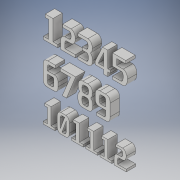
# Autodesk Inventor part: Number
Saved by Autodesk Inventor 2019 (Build 230136000, 136)
## iProperties
Created: 2019-03-23
Part Number: Number
Material: 一般
Document SubType Name: Modeling
Designer: j13tw
Density: 1 g/cm^3
Appearance: 預設
Author: j13tw
Autodesk Inventor part; units mm, degrees
ref_plane "YZ Plane" through (0, 0, 0) normal (1, 0, 0) x (0, 1, 0)
ref_plane "XZ Plane" through (0, 0, 0) normal (0, 1, 0) x (-1, 0, 0)
ref_plane "XY Plane" through (0, 0, 0) normal (0, 0, 1) x (1, 0, 0)
sketch "草圖3" plane through (0, 0, 0) normal (0, 0, 1) x (1, 0, 0)
  line L0 (-66.3082, 4.0187) -> (-27.2106, 4.0187) construction
  line L1 (-27.2106, 4.0187) -> (-27.2106, -2.3169) construction
  line L2 (-27.2106, -2.3169) -> (-66.3082, -2.3169) construction
  line L3 (-66.3082, -2.3169) -> (-66.3082, 4.0187) construction
  line L4 (-63.371, 4.0187) -> (-63.371, -1.3337)
  line L5 (-63.371, -1.3337) -> (-62.0793, -1.3337)
  line L6 (-62.0793, -1.3337) -> (-62.0793, -2.0813)
  line L7 (-62.0793, -2.0813) -> (-65.9322, -2.0813)
  line L8 (-65.9322, -2.0813) -> (-65.9322, -1.3337)
  line L9 (-65.9322, -1.3337) -> (-64.5344, -1.3337)
  line L10 (-64.5344, -1.3337) -> (-64.5344, 3.2401)
  line L11 (-64.5344, 3.2401) -> (-65.4324, 3.2401)
  line L12 (-65.4324, 3.2401) -> (-65.4324, 4.0187)
  line L13 (-65.4324, 4.0187) -> (-63.371, 4.0187)
  spline S0 degree 2 poles (-58.5892, 4.0187) (-58.3326, 4.0187) (-57.9036, 3.7577) (-57.5939, 3.2888) (-57.4303, 2.6695) (-57.4303, 2.3112) knots 0 0 0 1 2 3 4 4 4
  spline S1 degree 2 poles (-57.4303, 2.3112) (-57.4303, 1.9573) (-57.5939, 1.3557) (-57.8947, 0.909) (-58.3282, 0.6612) (-58.5892, 0.6612) knots 0 0 0 1 2 3 4 4 4
  line L14 (-58.5892, 0.6612) -> (-59.7482, 0.6612)
  spline S2 degree 2 poles (-59.7482, 0.6612) (-60.2126, 0.6612) (-60.2126, -0.2456) knots 0 0 0 1 1 1
  line L15 (-60.2126, -0.2456) -> (-60.2126, -1.3337)
  line L16 (-60.2126, -1.3337) -> (-57.4037, -1.3337)
  line L17 (-57.4037, -1.3337) -> (-57.4037, -2.0813)
  line L18 (-57.4037, -2.0813) -> (-61.3627, -2.0813)
  line L19 (-61.3627, -2.0813) -> (-61.3627, -0.2456)
  spline S3 degree 2 poles (-61.3627, -0.2456) (-61.3627, 0.1083) (-61.2123, 0.7188) (-60.916, 1.1655) (-60.5002, 1.4221) (-60.2303, 1.4221) knots 0 0 0 1 2 3 4 4 4
  line L20 (-60.2303, 1.4221) -> (-59.0891, 1.4221)
  spline S4 degree 2 poles (-59.0891, 1.4221) (-58.8413, 1.4221) (-58.545, 1.9441) (-58.545, 2.3378) knots 0 0 0 1 2 2 2
  spline S5 degree 2 poles (-58.545, 2.3378) (-58.545, 2.727) (-58.8413, 3.2578) (-59.0891, 3.2578) knots 0 0 0 1 2 2 2
  line L21 (-59.0891, 3.2578) -> (-60.7965, 3.2578)
  line L22 (-60.7965, 3.2578) -> (-60.7965, 4.0187)
  line L23 (-60.7965, 4.0187) -> (-58.5892, 4.0187)
  spline S6 degree 2 poles (-54.0817, 4.0187) (-53.8207, 4.0187) (-53.3828, 3.7621) (-53.0731, 3.3109) (-52.905, 2.7005) (-52.905, 2.3422) knots 0 0 0 1 2 3 4 4 4
  spline S7 degree 2 poles (-52.905, 2.3422) (-52.905, 1.4752) (-53.4181, 1.0771) knots 0 0 0 1 1 1
  spline S8 degree 2 poles (-53.4181, 1.0771) (-53.2899, 0.993) (-53.0643, 0.6745) (-52.8962, 0.2764) (-52.8077, -0.1615) (-52.8077, -0.3739) knots 0 0 0 1 2 3 4 4 4
  spline S9 degree 2 poles (-52.8077, -0.3739) (-52.8077, -0.7366) (-52.9802, -1.3559) (-53.281, -1.8159) (-53.7189, -2.0813) (-53.9755, -2.0813) knots 0 0 0 1 2 3 4 4 4
  line L24 (-53.9755, -2.0813) -> (-56.749, -2.0813)
  line L25 (-56.749, -2.0813) -> (-56.749, -1.3337)
  line L26 (-56.749, -1.3337) -> (-54.4665, -1.3337)
  spline S10 degree 2 poles (-54.4665, -1.3337) (-54.2276, -1.3337) (-53.9313, -0.7808) (-53.9313, -0.3385) knots 0 0 0 1 2 2 2
  spline S11 degree 2 poles (-53.9313, -0.3385) (-53.9313, -0.135) (-54.0065, 0.2233) (-54.1524, 0.4843) (-54.3471, 0.6391) (-54.4665, 0.6391) knots 0 0 0 1 2 3 4 4 4
  line L27 (-54.4665, 0.6391) -> (-55.5768, 0.6391)
  line L28 (-55.5768, 0.6391) -> (-55.5768, 1.4)
  line L29 (-55.5768, 1.4) -> (-54.5683, 1.4)
  spline S12 degree 2 poles (-54.5683, 1.4) (-54.3117, 1.4) (-54.0286, 1.86) (-54.0286, 2.3112) knots 0 0 0 1 2 2 2
  spline S13 degree 2 poles (-54.0286, 2.3112) (-54.0286, 2.7668) (-54.3117, 3.2578) (-54.5683, 3.2578) knots 0 0 0 1 2 2 2
  line L30 (-54.5683, 3.2578) -> (-56.749, 3.2578)
  line L31 (-56.749, 3.2578) -> (-56.749, 4.0187)
  line L32 (-56.749, 4.0187) -> (-54.0817, 4.0187)
  line L33 (-48.7912, 4.0187) -> (-48.7912, -0.2544)
  line L34 (-48.7912, -0.2544) -> (-48.163, -0.2544)
  line L35 (-48.163, -0.2544) -> (-48.163, -0.9843)
  line L36 (-48.163, -0.9843) -> (-48.7912, -0.9843)
  line L37 (-48.7912, -0.9843) -> (-48.7912, -2.0813)
  line L38 (-48.7912, -2.0813) -> (-49.8705, -2.0813)
  line L39 (-49.8705, -2.0813) -> (-49.8705, -0.9843)
  line L40 (-49.8705, -0.9843) -> (-52.1574, -0.9843)
  line L41 (-52.1574, -0.9843) -> (-52.1574, -0.1615)
  line L42 (-52.1574, -0.1615) -> (-50.2244, 4.0187)
  line L43 (-50.2244, 4.0187) -> (-48.7912, 4.0187)
  line L44 (-51.3214, -0.2544) -> (-49.8705, -0.2544)
  line L45 (-49.8705, -0.2544) -> (-49.8705, 2.8818)
  line L46 (-49.8705, 2.8818) -> (-51.3214, -0.2544)
  line L47 (-44.0182, 4.0187) -> (-44.0182, 3.2578)
  line L48 (-44.0182, 3.2578) -> (-46.4202, 3.2578)
  line L49 (-46.4202, 3.2578) -> (-46.4202, 1.7008)
  line L50 (-46.4202, 1.7008) -> (-44.695, 1.7008)
  spline S14 degree 2 poles (-44.695, 1.7008) (-44.434, 1.7008) (-44.0094, 1.4132) (-43.7174, 0.9311) (-43.5582, 0.2897) (-43.5582, -0.0598) knots 0 0 0 1 2 3 4 4 4
  spline S15 degree 2 poles (-43.5582, -0.0598) (-43.5582, -0.4358) (-43.7395, -1.1657) (-44.0536, -1.7319) (-44.5004, -2.0813) (-44.7569, -2.0813) knots 0 0 0 1 2 3 4 4 4
  line L51 (-44.7569, -2.0813) -> (-47.5437, -2.0813)
  line L52 (-47.5437, -2.0813) -> (-47.5437, -1.3337)
  line L53 (-47.5437, -1.3337) -> (-45.2568, -1.3337)
  spline S16 degree 2 poles (-45.2568, -1.3337) (-45.1197, -1.3337) (-44.9073, -1.1126) (-44.7658, -0.7587) (-44.6817, -0.3075) (-44.6817, -0.0731) knots 0 0 0 1 2 3 4 4 4
  spline S17 degree 2 poles (-44.6817, -0.0731) (-44.6817, 0.4047) (-44.925, 0.9399) (-45.1816, 0.9399) knots 0 0 0 1 2 2 2
  line L54 (-45.1816, 0.9399) -> (-47.5437, 0.9399)
  line L55 (-47.5437, 0.9399) -> (-47.5437, 4.0187)
  line L56 (-47.5437, 4.0187) -> (-44.0182, 4.0187)
  line L57 (-62.7384, -6.4217) -> (-62.7384, -7.2046)
  line L58 (-62.7384, -7.2046) -> (-64.3751, -7.2046)
  spline S18 degree 2 poles (-64.3751, -7.2046) (-64.6317, -7.2046) (-64.8263, -7.5364) (-64.8263, -8.0141) knots 0 0 0 1 2 2 2
  line L59 (-64.8263, -8.0141) -> (-64.8263, -8.7705)
  line L60 (-64.8263, -8.7705) -> (-63.0171, -8.7705)
  spline S19 degree 2 poles (-63.0171, -8.7705) (-62.5305, -8.7705) (-62.0174, -9.4341) (-62.0174, -10.0091) knots 0 0 0 1 2 2 2
  line L61 (-62.0174, -10.0091) -> (-62.0174, -11.0354)
  spline S20 degree 2 poles (-62.0174, -11.0354) (-62.0174, -11.4645) (-62.1545, -12.0395) (-62.4553, -12.3801) (-62.9331, -12.5217) (-63.2781, -12.5217) knots 0 0 0 1 2 3 4 4 4
  line L62 (-63.2781, -12.5217) -> (-64.729, -12.5217)
  spline S21 degree 2 poles (-64.729, -12.5217) (-65.0696, -12.5217) (-65.5474, -12.3801) (-65.8393, -12.0395) (-65.9764, -11.4645) (-65.9764, -11.0354) knots 0 0 0 1 2 3 4 4 4
  line L63 (-65.9764, -11.0354) -> (-65.9764, -7.8991)
  spline S22 degree 2 poles (-65.9764, -7.8991) (-65.9764, -7.47) (-65.8393, -6.9038) (-65.5474, -6.5632) (-65.0696, -6.4217) (-64.729, -6.4217) knots 0 0 0 1 2 3 4 4 4
  line L64 (-64.729, -6.4217) -> (-62.7384, -6.4217)
  spline S23 degree 2 poles (-64.8263, -10.9602) (-64.8263, -11.199) (-64.7821, -11.5175) (-64.6759, -11.6989) (-64.5034, -11.7741) (-64.3751, -11.7741) knots 0 0 0 1 2 3 4 4 4
  line L65 (-64.3751, -11.7741) -> (-63.5966, -11.7741)
  spline S24 degree 2 poles (-63.5966, -11.7741) (-63.371, -11.7741) (-63.1587, -11.4954) (-63.1587, -11.1238) knots 0 0 0 1 2 2 2
  line L66 (-63.1587, -11.1238) -> (-63.1587, -10.0357)
  spline S25 degree 2 poles (-63.1587, -10.0357) (-63.1587, -9.5225) (-63.4108, -9.5225) knots 0 0 0 1 1 1
  line L67 (-63.4108, -9.5225) -> (-64.8263, -9.5225)
  line L68 (-64.8263, -9.5225) -> (-64.8263, -10.9602)
  line L69 (-57.3241, -6.4217) -> (-59.7747, -12.5217)
  line L70 (-59.7747, -12.5217) -> (-60.9248, -12.5217)
  line L71 (-60.9248, -12.5217) -> (-58.7131, -7.1825)
  line L72 (-58.7131, -7.1825) -> (-61.4512, -7.1825)
  line L73 (-61.4512, -7.1825) -> (-61.4512, -6.4217)
  line L74 (-61.4512, -6.4217) -> (-57.3241, -6.4217)
  spline S26 degree 2 poles (-55.5326, -12.5217) (-56.143, -12.5217) (-56.78, -11.6547) (-56.78, -10.739) knots 0 0 0 1 2 2 2
  spline S27 degree 2 poles (-56.78, -10.739) (-56.78, -10.1286) (-56.5013, -9.4429) (-56.2182, -9.2616) knots 0 0 0 1 2 2 2
  spline S28 degree 2 poles (-56.2182, -9.2616) (-56.3244, -9.1598) (-56.4925, -8.9519) (-56.6119, -8.6644) (-56.6827, -8.2707) (-56.6827, -7.9964) knots 0 0 0 1 2 3 4 4 4
  spline S29 degree 2 poles (-56.6827, -7.9964) (-56.6827, -7.2444) (-56.0678, -6.4217) (-55.4264, -6.4217) knots 0 0 0 1 2 2 2
  line L75 (-55.4264, -6.4217) -> (-54.1215, -6.4217)
  spline S30 degree 2 poles (-54.1215, -6.4217) (-53.4801, -6.4217) (-52.8829, -7.2046) (-52.8829, -7.9964) knots 0 0 0 1 2 2 2
  spline S31 degree 2 poles (-52.8829, -7.9964) (-52.8829, -8.2707) (-52.9493, -8.6644) (-53.0731, -8.9519) (-53.2279, -9.1598) (-53.3297, -9.2616) knots 0 0 0 1 2 3 4 4 4
  spline S32 degree 2 poles (-53.3297, -9.2616) (-53.0554, -9.4429) (-52.7767, -10.1286) (-52.7767, -10.739) knots 0 0 0 1 2 2 2
  spline S33 degree 2 poles (-52.7767, -10.739) (-52.7767, -12.5217) (-54.0242, -12.5217) knots 0 0 0 1 1 1
  line L76 (-54.0242, -12.5217) -> (-55.5326, -12.5217)
  spline S34 degree 2 poles (-55.1256, -9.7658) (-55.3689, -9.7658) (-55.6697, -10.1949) (-55.6697, -10.7036) knots 0 0 0 1 2 2 2
  spline S35 degree 2 poles (-55.6697, -10.7036) (-55.6697, -11.2477) (-55.3689, -11.7741) (-55.1256, -11.7741) knots 0 0 0 1 2 2 2
  line L77 (-55.1256, -11.7741) -> (-54.4311, -11.7741)
  spline S36 degree 2 poles (-54.4311, -11.7741) (-54.1834, -11.7741) (-53.8738, -11.2477) (-53.8738, -10.7036) knots 0 0 0 1 2 2 2
  spline S37 degree 2 poles (-53.8738, -10.7036) (-53.8738, -10.1949) (-54.1834, -9.7658) (-54.4311, -9.7658) knots 0 0 0 1 2 2 2
  line L78 (-54.4311, -9.7658) -> (-55.1256, -9.7658)
  spline S38 degree 2 poles (-55.1256, -7.1825) (-55.3689, -7.1825) (-55.652, -7.6602) (-55.652, -8.0982) knots 0 0 0 1 2 2 2
  spline S39 degree 2 poles (-55.652, -8.0982) (-55.652, -8.5361) (-55.3689, -9.005) (-55.1256, -9.005) knots 0 0 0 1 2 2 2
  line L79 (-55.1256, -9.005) -> (-54.4311, -9.005)
  spline S40 degree 2 poles (-54.4311, -9.005) (-54.1834, -9.005) (-53.8959, -8.5361) (-53.8959, -8.0982) knots 0 0 0 1 2 2 2
  spline S41 degree 2 poles (-53.8959, -8.0982) (-53.8959, -7.6602) (-54.1834, -7.1825) (-54.4311, -7.1825) knots 0 0 0 1 2 2 2
  line L80 (-54.4311, -7.1825) -> (-55.1256, -7.1825)
  spline S42 degree 2 poles (-49.4458, -6.3996) (-49.1008, -6.3996) (-48.6142, -6.55) (-48.3134, -6.8906) (-48.1763, -7.4612) (-48.1763, -7.877) knots 0 0 0 1 2 3 4 4 4
  line L81 (-48.1763, -7.877) -> (-48.1763, -11.0354)
  spline S43 degree 2 poles (-48.1763, -11.0354) (-48.1763, -11.4645) (-48.3134, -12.0307) (-48.6142, -12.3801) (-49.1008, -12.5217) (-49.4458, -12.5217) knots 0 0 0 1 2 3 4 4 4
  line L82 (-49.4458, -12.5217) -> (-51.7859, -12.5217)
  line L83 (-51.7859, -12.5217) -> (-51.7859, -11.7741)
  line L84 (-51.7859, -11.7741) -> (-49.8263, -11.7741)
  spline S44 degree 2 poles (-49.8263, -11.7741) (-49.698, -11.7741) (-49.521, -11.7077) (-49.4105, -11.5264) (-49.3618, -11.2167) (-49.3618, -10.9734) knots 0 0 0 1 2 3 4 4 4
  line L85 (-49.3618, -10.9734) -> (-49.3618, -10.0976)
  line L86 (-49.3618, -10.0976) -> (-51.1445, -10.0976)
  spline S45 degree 2 poles (-51.1445, -10.0976) (-51.6443, -10.0976) (-52.1442, -9.412) (-52.1442, -8.859) knots 0 0 0 1 2 2 2
  line L87 (-52.1442, -8.859) -> (-52.1442, -7.877)
  spline S46 degree 2 poles (-52.1442, -7.877) (-52.1442, -7.4612) (-52.0159, -6.8906) (-51.7195, -6.55) (-51.2418, -6.3996) (-50.8967, -6.3996) knots 0 0 0 1 2 3 4 4 4
  line L88 (-50.8967, -6.3996) -> (-49.4458, -6.3996)
  spline S47 degree 2 poles (-50.534, -7.1825) (-50.6756, -7.1825) (-50.8569, -7.3019) (-50.9587, -7.585) (-50.9941, -8.0362) (-50.9941, -8.368) knots 0 0 0 1 2 3 4 4 4
  spline S48 degree 2 poles (-50.9941, -8.368) (-50.9941, -8.8679) (-50.8967, -9.3412) (-50.7287, -9.3412) knots 0 0 0 1 2 2 2
  line L89 (-50.7287, -9.3412) -> (-49.3618, -9.3412)
  line L90 (-49.3618, -9.3412) -> (-49.3618, -7.9964)
  spline S49 degree 2 poles (-49.3618, -7.9964) (-49.3618, -7.5231) (-49.5697, -7.1825) (-49.8263, -7.1825) knots 0 0 0 1 2 2 2
  line L91 (-49.8263, -7.1825) -> (-50.534, -7.1825)
  line L92 (-63.9007, -16.5717) -> (-63.9007, -20.9589)
  line L93 (-63.9007, -20.9589) -> (-62.8419, -20.9589)
  line L94 (-62.8419, -20.9589) -> (-62.8419, -21.5717)
  line L95 (-62.8419, -21.5717) -> (-66, -21.5717)
  line L96 (-66, -21.5717) -> (-66, -20.9589)
  line L97 (-66, -20.9589) -> (-64.8543, -20.9589)
  line L98 (-64.8543, -20.9589) -> (-64.8543, -17.2098)
  line L99 (-64.8543, -17.2098) -> (-65.5903, -17.2098)
  line L100 (-65.5903, -17.2098) -> (-65.5903, -16.5717)
  line L101 (-65.5903, -16.5717) -> (-63.9007, -16.5717)
  spline S50 degree 2 poles (-59.9594, -16.5717) (-59.7527, -16.5717) (-59.401, -16.782) (-59.1472, -17.1518) (-59.0058, -17.6522) (-59.0058, -17.9459) knots 0 0 0 1 2 3 4 4 4
  line L102 (-59.0058, -17.9459) -> (-59.0058, -20.2156)
  spline S51 degree 2 poles (-59.0058, -20.2156) (-59.0058, -20.4948) (-59.14, -20.9916) (-59.3938, -21.3614) (-59.7491, -21.5717) (-59.9594, -21.5717) knots 0 0 0 1 2 3 4 4 4
  line L103 (-59.9594, -21.5717) -> (-61.3118, -21.5717)
  spline S52 degree 2 poles (-61.3118, -21.5717) (-61.5294, -21.5717) (-61.8811, -21.3614) (-62.1313, -20.9916) (-62.2727, -20.4948) (-62.2727, -20.2156) knots 0 0 0 1 2 3 4 4 4
  line L104 (-62.2727, -20.2156) -> (-62.2727, -17.9459)
  spline S53 degree 2 poles (-62.2727, -17.9459) (-62.2727, -17.6522) (-62.1313, -17.1518) (-61.8775, -16.782) (-61.5221, -16.5717) (-61.3118, -16.5717) knots 0 0 0 1 2 3 4 4 4
  line L105 (-61.3118, -16.5717) -> (-59.9594, -16.5717)
  line L106 (-61.4242, -20.3643) -> (-60.2785, -17.1953)
  line L107 (-60.2785, -17.1953) -> (-60.9783, -17.1953)
  spline S54 degree 2 poles (-60.9783, -17.1953) (-61.0834, -17.1953) (-61.2466, -17.3186) (-61.3626, -17.5253) (-61.4242, -17.7972) (-61.4242, -17.9459) knots 0 0 0 1 2 3 4 4 4
  line L108 (-61.4242, -17.9459) -> (-61.4242, -20.3643)
  line L109 (-60.9674, -20.9589) -> (-60.2966, -20.9589)
  spline S55 degree 2 poles (-60.2966, -20.9589) (-60.1987, -20.9589) (-60.0247, -20.8357) (-59.9086, -20.6326) (-59.8398, -20.3643) (-59.8398, -20.2156) knots 0 0 0 1 2 3 4 4 4
  line L110 (-59.8398, -20.2156) -> (-59.8398, -17.8226)
  line L111 (-59.8398, -17.8226) -> (-60.9674, -20.9589)
  line L112 (-56.3372, -16.5717) -> (-56.3372, -20.9589)
  line L113 (-56.3372, -20.9589) -> (-55.2785, -20.9589)
  line L114 (-55.2785, -20.9589) -> (-55.2785, -21.5717)
  line L115 (-55.2785, -21.5717) -> (-58.4366, -21.5717)
  line L116 (-58.4366, -21.5717) -> (-58.4366, -20.9589)
  line L117 (-58.4366, -20.9589) -> (-57.2908, -20.9589)
  line L118 (-57.2908, -20.9589) -> (-57.2908, -17.2098)
  line L119 (-57.2908, -17.2098) -> (-58.0268, -17.2098)
  line L120 (-58.0268, -17.2098) -> (-58.0268, -16.5717)
  line L121 (-58.0268, -16.5717) -> (-56.3372, -16.5717)
  line L122 (-52.5555, -16.5717) -> (-52.5555, -20.9589)
  line L123 (-52.5555, -20.9589) -> (-51.4967, -20.9589)
  line L124 (-51.4967, -20.9589) -> (-51.4967, -21.5717)
  line L125 (-51.4967, -21.5717) -> (-54.6548, -21.5717)
  line L126 (-54.6548, -21.5717) -> (-54.6548, -20.9589)
  line L127 (-54.6548, -20.9589) -> (-53.5091, -20.9589)
  line L128 (-53.5091, -20.9589) -> (-53.5091, -17.2098)
  line L129 (-53.5091, -17.2098) -> (-54.2451, -17.2098)
  line L130 (-54.2451, -17.2098) -> (-54.2451, -16.5717)
  line L131 (-54.2451, -16.5717) -> (-52.5555, -16.5717)
  line L132 (-48.7738, -16.5717) -> (-48.7738, -20.9589)
  line L133 (-48.7738, -20.9589) -> (-47.715, -20.9589)
  line L134 (-47.715, -20.9589) -> (-47.715, -21.5717)
  line L135 (-47.715, -21.5717) -> (-50.8731, -21.5717)
  line L136 (-50.8731, -21.5717) -> (-50.8731, -20.9589)
  line L137 (-50.8731, -20.9589) -> (-49.7274, -20.9589)
  line L138 (-49.7274, -20.9589) -> (-49.7274, -17.2098)
  line L139 (-49.7274, -17.2098) -> (-50.4634, -17.2098)
  line L140 (-50.4634, -17.2098) -> (-50.4634, -16.5717)
  line L141 (-50.4634, -16.5717) -> (-48.7738, -16.5717)
  spline S56 degree 2 poles (-44.8543, -16.5717) (-44.644, -16.5717) (-44.2923, -16.7856) (-44.0384, -17.17) (-43.9043, -17.6776) (-43.9043, -17.9713) knots 0 0 0 1 2 3 4 4 4
  spline S57 degree 2 poles (-43.9043, -17.9713) (-43.9043, -18.2613) (-44.0384, -18.7544) (-44.285, -19.1206) (-44.6403, -19.3237) (-44.8543, -19.3237) knots 0 0 0 1 2 3 4 4 4
  line L142 (-44.8543, -19.3237) -> (-45.8042, -19.3237)
  spline S58 degree 2 poles (-45.8042, -19.3237) (-46.1849, -19.3237) (-46.1849, -20.067) knots 0 0 0 1 1 1
  line L143 (-46.1849, -20.067) -> (-46.1849, -20.9589)
  line L144 (-46.1849, -20.9589) -> (-43.8825, -20.9589)
  line L145 (-43.8825, -20.9589) -> (-43.8825, -21.5717)
  line L146 (-43.8825, -21.5717) -> (-47.1276, -21.5717)
  line L147 (-47.1276, -21.5717) -> (-47.1276, -20.067)
  spline S59 degree 2 poles (-47.1276, -20.067) (-47.1276, -19.7769) (-47.0044, -19.2766) (-46.7614, -18.9103) (-46.4206, -18.7) (-46.1994, -18.7) knots 0 0 0 1 2 3 4 4 4
  line L148 (-46.1994, -18.7) -> (-45.264, -18.7)
  spline S60 degree 2 poles (-45.264, -18.7) (-45.0609, -18.7) (-44.818, -18.2722) (-44.818, -17.9495) knots 0 0 0 1 2 2 2
  spline S61 degree 2 poles (-44.818, -17.9495) (-44.818, -17.6304) (-45.0609, -17.1953) (-45.264, -17.1953) knots 0 0 0 1 2 2 2
  line L149 (-45.264, -17.1953) -> (-46.6635, -17.1953)
  line L150 (-46.6635, -17.1953) -> (-46.6635, -16.5717)
  line L151 (-46.6635, -16.5717) -> (-44.8543, -16.5717)
  constraints: 2 other
extrude "擠出3" add sketch "草圖3" along normal blind 2.5
